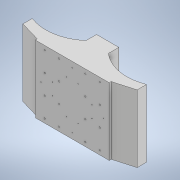
# Autodesk Inventor part: chassis
Saved by Autodesk Inventor 2020 (Build 240168000, 168)
## iProperties
Created: 2024-02-01
Part Number: chassis
Material: Générique
Document SubType Name: Modeling
Designer: Stark
Density: 1 g/cm^3
Appearance: Par défaut
Author: Stark
Autodesk Inventor part; units mm, degrees
ref_plane "YZ Plane" through (0, 0, 0) normal (1, 0, 0) x (0, 1, 0)
ref_plane "XZ Plane" through (0, 0, 0) normal (0, 1, 0) x (-1, 0, 0)
ref_plane "XY Plane" through (0, 0, 0) normal (0, 0, 1) x (1, 0, 0)
sketch "Esquisse4" plane through (0, 0, 0) normal (0, 1, 0) x (-1, 0, 0)
  line L0 (0, 0) -> (-562.5, 0)
  line L1 (-562.5, 0) -> (-562.5, -30)
  line L2 (-562.5, -30) -> (-870, -118.564948)
  line L3 (-870, -118.564948) -> (-870, -258.564948)
  line L4 (-870, -258.564948) -> (-860, -258.564948)
  line L5 (-170, -380) -> (-170, -540)
  line L6 (-170, -540) -> (0, -540)
  line L7 (0, -540) -> (0, 0)
  circle A0 centre (-616.322156, -895) radius 300 construction
  arc A1 (-170, -380) -> (-860, -258.564948) centre (-616.322156, -895) ccw
  point P0 (-870, -248.564948)
  dimension "d54" = 562.5
  dimension "d63" = 540
  dimension "d64" = 870
  dimension "d65" = 600
  dimension "d66" = 170
  dimension "d67" = 160
  dimension "d68" = 140
  dimension "d69" = 10
  dimension "d70" = 30
  dimension "d72" = 106.067
  dimension "d73" = 895
  constraints: 16 end point, 3 coincident, 3 horizontal, 3 vertical, 2 centre point, 2 point on circle
  measures "d54" distance of L0.start L0.end
  measures "d63" distance of L7.start L0.start
  measures "d64" distance between parallel lines of L3 L7
  measures "d65" diameter of A0
  measures "d66" distance of L5.end L7.start
  measures "d67" distance of L5.start L5.end
  measures "d68" distance of L3.start L4.start
  measures "d69" distance of L4.start L4.end
  measures "d70" distance of L0.end L1.end
  measures "d72" angle of L2 L1
  measures "d73" distance from line of A0.centre L0
sketch "Esquisse4 outline for Extrusion2" plane through (0, 0, 0) normal (0, 1, 0) x (-1, 0, 0)
  line L0 (-170, -380) -> (-170, -540)
  arc A0 (-860, -258.564948) -> (-170, -380) centre (-616.322156, -895) cw
  line L1 (-870, -258.564948) -> (-860, -258.564948)
  line L2 (-870, -118.564948) -> (-870, -258.564948)
  line L3 (-562.5, -30) -> (-870, -118.564948)
  line L4 (-562.5, 0) -> (-562.5, -30)
  line L5 (0, 0) -> (-562.5, 0)
  line L6 (0, -540) -> (0, 0)
  line L7 (-170, -540) -> (0, -540)
extrude "Extrusion2" add sketch "Esquisse4 outline for Extrusion2" against normal blind 512.5
sketch "Esquisse6" plane through (0, 0, 0) normal (0, 0, 1) x (1, 0, 0)
  line L0 (0, 0) -> (562.5, 0) projected
  line L1 (0, 0) -> (0, -512.5) projected
  line L2 (562.5, 0) -> (562.5, -512.5) projected
  point P0 (300, -90)
  point P1 (90, -262.5)
  point P2 (477.5, 0)
  point P3 (0, -427.5)
  dimension "d96" = 85
  dimension "d97" = 85
  dimension "d98" = 90
  dimension "d99" = 90
  dimension "d100" = 262.5
  dimension "d101" = 262.5
  constraints: 2 point on line
  measures "d96" distance of L0.end point (477.5, 0)
  measures "d97" distance of L1.end point (0, -427.5)
  measures "d98" distance from line of L1 point (90, -262.5)
  measures "d99" distance from line of L0 point (300, -90)
  measures "d100" distance from line of L2 point (300, -90)
  measures "d101" distance from line of L0 point (90, -262.5)
hole "Perçage4" at (90, -262.5, 0) at (0, -427.5, 0) at (300, -90, 0) at (477.5, 0, 0) direction (0, 0, -1) diameter 10 depth 40 tip angle 118
sketch "Esquisse7" plane through (0, -512.5, 0) normal (0, 0, 1) x (1, 0, 0)
  line L0 (200, 362.5) -> (420, 362.5) construction
  line L1 (420, 362.5) -> (420, 62.5) construction
  line L2 (420, 62.5) -> (200, 62.5) construction
  line L3 (200, 62.5) -> (200, 362.5) construction
  line L4 (562.5, 0) -> (0, 0) construction
  line L5 (562.5, 512.5) -> (562.5, 0) construction
  point P0 (0, 512.5)
  dimension "d109" = 62.5
  dimension "d110" = 142.5
  dimension "d111" = 300
  dimension "d112" = 220
  constraints: 8 end point, 2 coincident, 2 parallel, 1 horizontal, 1 perpendicular
  measures "d109" distance from line of L4 point (420, 62.5)
  measures "d110" distance between parallel lines of L5 L1
  measures "d111" distance of L0.end L1.end
  measures "d112" distance of L0.start L0.end
hole "Perçage5" at (420, -450, 0) at (200, -150, 0) at (200, -450, 0) at (420, -150, 0) direction (0, 0, -1) diameter 20 depth 40 tip angle 118
mirror "Symétrie3" about plane through (435, 0, -270) normal (0, 1, 0) of "Extrusion2", "Perçage4", "Perçage5"
mirror "Symétrie4" about plane through (0, 0, 0) normal (-1, 0, 0) of "Extrusion2", "Perçage4", "Perçage5", "Symétrie3"
